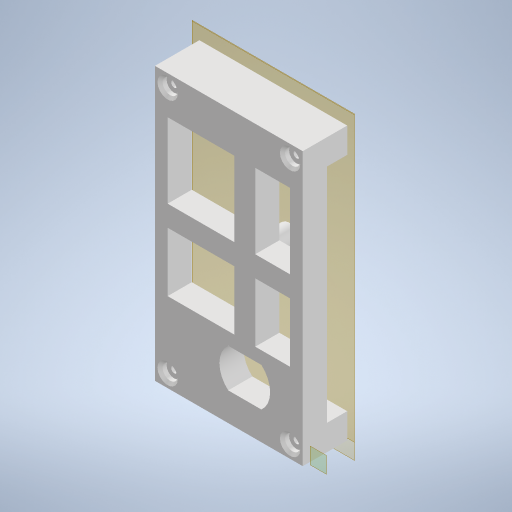
# Autodesk Inventor part: housingFront
Saved by Autodesk Inventor 2023 (Build 270158000, 158)
## iProperties
Created: 2023-03-11
Part Number: housingFront
Material: Generic
Document SubType Name: Modeling
Designer: shrey
Density: 1 g/cm^3
Appearance: Default
Author: shrey
Autodesk Inventor part; units mm, degrees
(part 1 of 2)
ref_plane "YZ Plane" through (0, 0, 0) normal (1, 0, 0) x (0, 1, 0)
ref_plane "XZ Plane" through (0, 0, 0) normal (0, 1, 0) x (-1, 0, 0)
ref_plane "XY Plane" through (0, 0, 0) normal (0, 0, 1) x (1, 0, 0)
ref_plane "Work Plane1" through (29.0854, -74.8946, 2) normal (0, 0, 1) x (1, 0, 0)
ref_plane "Work Plane2" through (29.0854, -80.3446, 2) normal (0, 0, 1) x (1, 0, 0)
sketch "Sketch3" plane through (29.0854, -80.3446, 2) normal (0, 0, 1) x (1, 0, 0)
  line L0 (29.0856, -48.6611) -> (29.0856, 58.6611) construction
  line L1 (29.0856, 58.6611) -> (-29.0856, 58.6611) construction
  line L2 (-29.0856, 58.6611) -> (-29.0856, -48.6611) construction
  line L3 (-29.0856, -48.6611) -> (29.0856, -48.6611) construction
  line L4 (29.0856, -48.6611) -> (-29.0856, -48.6611)
  line L5 (-29.0856, -48.6611) -> (-29.0856, 58.6611)
  line L6 (-29.0856, 58.6611) -> (29.0856, 58.6611)
  line L7 (29.0856, 58.6611) -> (29.0856, -48.6611)
  line L8 (29.0856, 48.6611) -> (-29.0856, 48.6611)
  spline S0 degree 3 poles (-74.8819, 38.2677) (-74.7621, 38.4578) (-74.5823, 38.743) (-74.3613, 39.1343) (-74.2025, 39.4317) (-74.052, 39.7333) (-73.9102, 40.0391) (-73.7782, 40.3493) (-73.6568, 40.6638) (-73.5477, 40.9828) (-73.4518, 41.306) (-73.3893, 41.58) (-73.3442, 41.8001) (-73.2966, 41.962) (-73.2322, 42.118) (-73.1482, 42.2647) (-73.0598, 42.3744) (-72.9799, 42.4536) (-72.9123, 42.5041) (-72.8431, 42.5525) (-72.7668, 42.5886) (-72.6893, 42.6221) (-72.6072, 42.6419) (-72.5245, 42.6586) (-72.4119, 42.6626) (-72.2715, 42.66) (-72.1312, 42.6626) (-72.0186, 42.6586) (-71.9359, 42.6419) (-71.8538, 42.6221) (-71.7763, 42.5886) (-71.7, 42.5525) (-71.6308, 42.5041) (-71.5632, 42.4536) (-71.4833, 42.3744) (-71.3948, 42.2647) (-71.3109, 42.118) (-71.2465, 41.962) (-71.1988, 41.8001) (-71.1538, 41.58) (-71.0913, 41.306) (-70.9954, 40.9828) (-70.8863, 40.6638) (-70.7649, 40.3493) (-70.6329, 40.0391) (-70.4911, 39.7333) (-70.3406, 39.4317) (-70.1818, 39.1343) (-69.9608, 38.743) (-69.781, 38.4578) (-69.6612, 38.2677) knots -1.0784 -1.0784 -1.0784 -1.0784 -1.010995 -0.977291 -0.943586 -0.909882 -0.876178 -0.842474 -0.80877 -0.775067 -0.741365 -0.707665 -0.690816 -0.67397 -0.657123 -0.640284 -0.623449 -0.615023 -0.606598 -0.598176 -0.589749 -0.581327 -0.572901 -0.564477 -0.556053 -0.5392 -0.522347 -0.513923 -0.505499 -0.497074 -0.488651 -0.480225 -0.471802 -0.463377 -0.454951 -0.438116 -0.421277 -0.40443 -0.387584 -0.370735 -0.337035 -0.303333 -0.26963 -0.235926 -0.202222 -0.168518 -0.134814 -0.101109 -0.067405 0 0 0 0 construction
  line L9 (-69.6612, 38.2677) -> (-68.5989, 38.2677) construction
  spline S1 degree 3 poles (-68.5989, 38.2677) (-68.4791, 38.4578) (-68.2993, 38.743) (-68.0783, 39.1343) (-67.9195, 39.4317) (-67.769, 39.7333) (-67.6272, 40.0391) (-67.4952, 40.3493) (-67.3738, 40.6638) (-67.2647, 40.9828) (-67.1688, 41.306) (-67.1063, 41.58) (-67.0612, 41.8001) (-67.0136, 41.962) (-66.9492, 42.118) (-66.8652, 42.2647) (-66.7768, 42.3744) (-66.6969, 42.4536) (-66.6293, 42.5041) (-66.5601, 42.5525) (-66.4838, 42.5886) (-66.4063, 42.6221) (-66.3242, 42.6419) (-66.2415, 42.6586) (-66.1289, 42.6626) (-65.9885, 42.66) (-65.8482, 42.6626) (-65.7356, 42.6586) (-65.6529, 42.6419) (-65.5708, 42.6221) (-65.4933, 42.5886) (-65.417, 42.5525) (-65.3478, 42.5041) (-65.2802, 42.4536) (-65.2003, 42.3744) (-65.1118, 42.2647) (-65.0279, 42.118) (-64.9635, 41.962) (-64.9158, 41.8001) (-64.8708, 41.58) (-64.8083, 41.306) (-64.7124, 40.9828) (-64.6033, 40.6638) (-64.4819, 40.3493) (-64.3499, 40.0391) (-64.2081, 39.7333) (-64.0576, 39.4317) (-63.8988, 39.1343) (-63.6778, 38.743) (-63.498, 38.4578) (-63.3782, 38.2677) knots -1.0784 -1.0784 -1.0784 -1.0784 -1.010995 -0.977291 -0.943586 -0.909882 -0.876178 -0.842474 -0.80877 -0.775067 -0.741365 -0.707665 -0.690816 -0.67397 -0.657123 -0.640284 -0.623449 -0.615023 -0.606598 -0.598176 -0.589749 -0.581327 -0.572901 -0.564477 -0.556053 -0.5392 -0.522347 -0.513923 -0.505499 -0.497074 -0.488651 -0.480225 -0.471802 -0.463377 -0.454951 -0.438116 -0.421277 -0.40443 -0.387584 -0.370735 -0.337035 -0.303333 -0.26963 -0.235926 -0.202222 -0.168518 -0.134814 -0.101109 -0.067405 0 0 0 0 construction
  line L10 (-63.3782, 38.2677) -> (-62.3159, 38.2677) construction
  spline S2 degree 3 poles (-62.3159, 38.2677) (-62.1961, 38.4578) (-62.0163, 38.743) (-61.7953, 39.1343) (-61.6365, 39.4317) (-61.486, 39.7333) (-61.3442, 40.0391) (-61.2122, 40.3493) (-61.0908, 40.6638) (-60.9817, 40.9828) (-60.8858, 41.306) (-60.8233, 41.58) (-60.7782, 41.8001) (-60.7306, 41.962) (-60.6662, 42.118) (-60.5822, 42.2647) (-60.4938, 42.3744) (-60.4139, 42.4536) (-60.3463, 42.5041) (-60.2771, 42.5525) (-60.2008, 42.5886) (-60.1233, 42.6221) (-60.0412, 42.6419) (-59.9585, 42.6586) (-59.8459, 42.6626) (-59.7055, 42.66) (-59.5652, 42.6626) (-59.4526, 42.6586) (-59.3699, 42.6419) (-59.2878, 42.6221) (-59.2103, 42.5886) (-59.134, 42.5525) (-59.0648, 42.5041) (-58.9972, 42.4536) (-58.9173, 42.3744) (-58.8288, 42.2647) (-58.7449, 42.118) (-58.6805, 41.962) (-58.6328, 41.8001) (-58.5878, 41.58) (-58.5253, 41.306) (-58.4294, 40.9828) (-58.3203, 40.6638) (-58.1989, 40.3493) (-58.0669, 40.0391) (-57.9251, 39.7333) (-57.7746, 39.4317) (-57.6158, 39.1343) (-57.3948, 38.743) (-57.215, 38.4578) (-57.0952, 38.2677) knots -1.0784 -1.0784 -1.0784 -1.0784 -1.010995 -0.977291 -0.943586 -0.909882 -0.876178 -0.842474 -0.80877 -0.775067 -0.741365 -0.707665 -0.690816 -0.67397 -0.657123 -0.640284 -0.623449 -0.615023 -0.606598 -0.598176 -0.589749 -0.581327 -0.572901 -0.564477 -0.556053 -0.5392 -0.522347 -0.513923 -0.505499 -0.497074 -0.488651 -0.480225 -0.471802 -0.463377 -0.454951 -0.438116 -0.421277 -0.40443 -0.387584 -0.370735 -0.337035 -0.303333 -0.26963 -0.235926 -0.202222 -0.168518 -0.134814 -0.101109 -0.067405 0 0 0 0 construction
  line L11 (-57.0952, 38.2677) -> (-56.0329, 38.2677) construction
  spline S3 degree 3 poles (-56.0329, 38.2677) (-55.9131, 38.4578) (-55.7333, 38.743) (-55.5123, 39.1343) (-55.3535, 39.4317) (-55.203, 39.7333) (-55.0612, 40.0391) (-54.9292, 40.3493) (-54.8078, 40.6638) (-54.6987, 40.9828) (-54.6028, 41.306) (-54.5403, 41.58) (-54.4952, 41.8001) (-54.4476, 41.962) (-54.3832, 42.118) (-54.2992, 42.2647) (-54.2108, 42.3744) (-54.1309, 42.4536) (-54.0633, 42.5041) (-53.9941, 42.5525) (-53.9178, 42.5886) (-53.8403, 42.6221) (-53.7582, 42.6419) (-53.6755, 42.6586) (-53.5629, 42.6626) (-53.4225, 42.66) (-53.2822, 42.6626) (-53.1696, 42.6586) (-53.0869, 42.6419) (-53.0048, 42.6221) (-52.9273, 42.5886) (-52.851, 42.5525) (-52.7818, 42.5041) (-52.7142, 42.4536) (-52.6343, 42.3744) (-52.5458, 42.2647) (-52.4619, 42.118) (-52.3975, 41.962) (-52.3498, 41.8001) (-52.3048, 41.58) (-52.2423, 41.306) (-52.1464, 40.9828) (-52.0373, 40.6638) (-51.9159, 40.3493) (-51.7839, 40.0391) (-51.6421, 39.7333) (-51.4916, 39.4317) (-51.3328, 39.1343) (-51.1118, 38.743) (-50.932, 38.4578) (-50.8122, 38.2677) knots -1.0784 -1.0784 -1.0784 -1.0784 -1.010995 -0.977291 -0.943586 -0.909882 -0.876178 -0.842474 -0.80877 -0.775067 -0.741365 -0.707665 -0.690816 -0.67397 -0.657123 -0.640284 -0.623449 -0.615023 -0.606598 -0.598176 -0.589749 -0.581327 -0.572901 -0.564477 -0.556053 -0.5392 -0.522347 -0.513923 -0.505499 -0.497074 -0.488651 -0.480225 -0.471802 -0.463377 -0.454951 -0.438116 -0.421277 -0.40443 -0.387584 -0.370735 -0.337035 -0.303333 -0.26963 -0.235926 -0.202222 -0.168518 -0.134814 -0.101109 -0.067405 0 0 0 0 construction
  line L12 (-50.8122, 38.2677) -> (-49.7499, 38.2677) construction
  spline S4 degree 3 poles (-49.7499, 38.2677) (-49.6301, 38.4578) (-49.4503, 38.743) (-49.2293, 39.1343) (-49.0705, 39.4317) (-48.92, 39.7333) (-48.7782, 40.0391) (-48.6462, 40.3493) (-48.5248, 40.6638) (-48.4157, 40.9828) (-48.3198, 41.306) (-48.2573, 41.58) (-48.2122, 41.8001) (-48.1646, 41.962) (-48.1002, 42.118) (-48.0162, 42.2647) (-47.9278, 42.3744) (-47.8479, 42.4536) (-47.7803, 42.5041) (-47.7111, 42.5525) (-47.6348, 42.5886) (-47.5573, 42.6221) (-47.4752, 42.6419) (-47.3925, 42.6586) (-47.2799, 42.6626) (-47.1395, 42.66) (-46.9992, 42.6626) (-46.8866, 42.6586) (-46.8039, 42.6419) (-46.7218, 42.6221) (-46.6443, 42.5886) (-46.568, 42.5525) (-46.4988, 42.5041) (-46.4312, 42.4536) (-46.3513, 42.3744) (-46.2628, 42.2647) (-46.1789, 42.118) (-46.1145, 41.962) (-46.0668, 41.8001) (-46.0218, 41.58) (-45.9593, 41.306) (-45.8634, 40.9828) (-45.7543, 40.6638) (-45.6329, 40.3493) (-45.5009, 40.0391) (-45.3591, 39.7333) (-45.2086, 39.4317) (-45.0498, 39.1343) (-44.8288, 38.743) (-44.649, 38.4578) (-44.5292, 38.2677) knots -1.0784 -1.0784 -1.0784 -1.0784 -1.010995 -0.977291 -0.943586 -0.909882 -0.876178 -0.842474 -0.80877 -0.775067 -0.741365 -0.707665 -0.690816 -0.67397 -0.657123 -0.640284 -0.623449 -0.615023 -0.606598 -0.598176 -0.589749 -0.581327 -0.572901 -0.564477 -0.556053 -0.5392 -0.522347 -0.513923 -0.505499 -0.497074 -0.488651 -0.480225 -0.471802 -0.463377 -0.454951 -0.438116 -0.421277 -0.40443 -0.387584 -0.370735 -0.337035 -0.303333 -0.26963 -0.235926 -0.202222 -0.168518 -0.134814 -0.101109 -0.067405 0 0 0 0 construction
  line L13 (-44.5292, 38.2677) -> (-43.4669, 38.2677) construction
  spline S5 degree 3 poles (-43.4669, 38.2677) (-43.3471, 38.4578) (-43.1673, 38.743) (-42.9463, 39.1343) (-42.7875, 39.4317) (-42.637, 39.7333) (-42.4952, 40.0391) (-42.3632, 40.3493) (-42.2418, 40.6638) (-42.1327, 40.9828) (-42.0368, 41.306) (-41.9743, 41.58) (-41.9292, 41.8001) (-41.8816, 41.962) (-41.8172, 42.118) (-41.7332, 42.2647) (-41.6448, 42.3744) (-41.5649, 42.4536) (-41.4973, 42.5041) (-41.4281, 42.5525) (-41.3518, 42.5886) (-41.2743, 42.6221) (-41.1922, 42.6419) (-41.1095, 42.6586) (-40.9969, 42.6626) (-40.8565, 42.66) (-40.7162, 42.6626) (-40.6036, 42.6586) (-40.5209, 42.6419) (-40.4388, 42.6221) (-40.3613, 42.5886) (-40.285, 42.5525) (-40.2158, 42.5041) (-40.1482, 42.4536) (-40.0683, 42.3744) (-39.9798, 42.2647) (-39.8959, 42.118) (-39.8315, 41.962) (-39.7838, 41.8001) (-39.7388, 41.58) (-39.6763, 41.306) (-39.5804, 40.9828) (-39.4713, 40.6638) (-39.3499, 40.3493) (-39.2179, 40.0391) (-39.0761, 39.7333) (-38.9256, 39.4317) (-38.7668, 39.1343) (-38.5458, 38.743) (-38.366, 38.4578) (-38.2462, 38.2677) knots -1.0784 -1.0784 -1.0784 -1.0784 -1.010995 -0.977291 -0.943586 -0.909882 -0.876178 -0.842474 -0.80877 -0.775067 -0.741365 -0.707665 -0.690816 -0.67397 -0.657123 -0.640284 -0.623449 -0.615023 -0.606598 -0.598176 -0.589749 -0.581327 -0.572901 -0.564477 -0.556053 -0.5392 -0.522347 -0.513923 -0.505499 -0.497074 -0.488651 -0.480225 -0.471802 -0.463377 -0.454951 -0.438116 -0.421277 -0.40443 -0.387584 -0.370735 -0.337035 -0.303333 -0.26963 -0.235926 -0.202222 -0.168518 -0.134814 -0.101109 -0.067405 0 0 0 0 construction
  line L14 (-38.2462, 38.2677) -> (-37.1839, 38.2677) construction
  spline S6 degree 3 poles (-37.1839, 38.2677) (-37.0641, 38.4578) (-36.8843, 38.743) (-36.6633, 39.1343) (-36.5045, 39.4317) (-36.354, 39.7333) (-36.2122, 40.0391) (-36.0802, 40.3493) (-35.9588, 40.6638) (-35.8497, 40.9828) (-35.7538, 41.306) (-35.6913, 41.58) (-35.6462, 41.8001) (-35.5986, 41.962) (-35.5342, 42.118) (-35.4502, 42.2647) (-35.3618, 42.3744) (-35.2819, 42.4536) (-35.2143, 42.5041) (-35.1451, 42.5525) (-35.0688, 42.5886) (-34.9913, 42.6221) (-34.9092, 42.6419) (-34.8265, 42.6586) (-34.7139, 42.6626) (-34.5735, 42.66) (-34.4332, 42.6626) (-34.3206, 42.6586) (-34.2379, 42.6419) (-34.1558, 42.6221) (-34.0783, 42.5886) (-34.002, 42.5525) (-33.9328, 42.5041) (-33.8652, 42.4536) (-33.7853, 42.3744) (-33.6968, 42.2647) (-33.6129, 42.118) (-33.5485, 41.962) (-33.5008, 41.8001) (-33.4558, 41.58) (-33.3933, 41.306) (-33.2974, 40.9828) (-33.1883, 40.6638) (-33.0669, 40.3493) (-32.9349, 40.0391) (-32.7931, 39.7333) (-32.6426, 39.4317) (-32.4838, 39.1343) (-32.2628, 38.743) (-32.083, 38.4578) (-31.9632, 38.2677) knots -1.0784 -1.0784 -1.0784 -1.0784 -1.010995 -0.977291 -0.943586 -0.909882 -0.876178 -0.842474 -0.80877 -0.775067 -0.741365 -0.707665 -0.690816 -0.67397 -0.657123 -0.640284 -0.623449 -0.615023 -0.606598 -0.598176 -0.589749 -0.581327 -0.572901 -0.564477 -0.556053 -0.5392 -0.522347 -0.513923 -0.505499 -0.497074 -0.488651 -0.480225 -0.471802 -0.463377 -0.454951 -0.438116 -0.421277 -0.40443 -0.387584 -0.370735 -0.337035 -0.303333 -0.26963 -0.235926 -0.202222 -0.168518 -0.134814 -0.101109 -0.067405 0 0 0 0 construction
  line L15 (-31.9632, 38.2677) -> (-30.9009, 38.2677) construction
  spline S7 degree 3 poles (-30.9009, 38.2677) (-30.7811, 38.4578) (-30.6013, 38.743) (-30.3803, 39.1343) (-30.2215, 39.4317) (-30.071, 39.7333) (-29.9292, 40.0391) (-29.7972, 40.3493) (-29.6758, 40.6638) (-29.5667, 40.9828) (-29.4708, 41.306) (-29.4083, 41.58) (-29.3632, 41.8001) (-29.3156, 41.962) (-29.2512, 42.118) (-29.1672, 42.2647) (-29.0788, 42.3744) (-28.9989, 42.4536) (-28.9313, 42.5041) (-28.8621, 42.5525) (-28.7858, 42.5886) (-28.7083, 42.6221) (-28.6262, 42.6419) (-28.5435, 42.6586) (-28.4309, 42.6626) (-28.2905, 42.66) (-28.1502, 42.6626) (-28.0376, 42.6586) (-27.9549, 42.6419) (-27.8728, 42.6221) (-27.7953, 42.5886) (-27.719, 42.5525) (-27.6498, 42.5041) (-27.5822, 42.4536) (-27.5023, 42.3744) (-27.4138, 42.2647) (-27.3299, 42.118) (-27.2655, 41.962) (-27.2178, 41.8001) (-27.1728, 41.58) (-27.1103, 41.306) (-27.0144, 40.9828) (-26.9053, 40.6638) (-26.7839, 40.3493) (-26.6519, 40.0391) (-26.5101, 39.7333) (-26.3596, 39.4317) (-26.2008, 39.1343) (-25.9798, 38.743) (-25.8, 38.4578) (-25.6802, 38.2677) knots -1.0784 -1.0784 -1.0784 -1.0784 -1.010995 -0.977291 -0.943586 -0.909882 -0.876178 -0.842474 -0.80877 -0.775067 -0.741365 -0.707665 -0.690816 -0.67397 -0.657123 -0.640284 -0.623449 -0.615023 -0.606598 -0.598176 -0.589749 -0.581327 -0.572901 -0.564477 -0.556053 -0.5392 -0.522347 -0.513923 -0.505499 -0.497074 -0.488651 -0.480225 -0.471802 -0.463377 -0.454951 -0.438116 -0.421277 -0.40443 -0.387584 -0.370735 -0.337035 -0.303333 -0.26963 -0.235926 -0.202222 -0.168518 -0.134814 -0.101109 -0.067405 0 0 0 0 construction
  line L16 (-25.6802, 38.2677) -> (-24.6179, 38.2677) construction
  spline S8 degree 3 poles (-24.6179, 38.2677) (-24.4981, 38.4578) (-24.3183, 38.743) (-24.0973, 39.1343) (-23.9385, 39.4317) (-23.788, 39.7333) (-23.6462, 40.0391) (-23.5142, 40.3493) (-23.3928, 40.6638) (-23.2837, 40.9828) (-23.1878, 41.306) (-23.1253, 41.58) (-23.0802, 41.8001) (-23.0326, 41.962) (-22.9682, 42.118) (-22.8842, 42.2647) (-22.7958, 42.3744) (-22.7159, 42.4536) (-22.6483, 42.5041) (-22.5791, 42.5525) (-22.5028, 42.5886) (-22.4253, 42.6221) (-22.3432, 42.6419) (-22.2605, 42.6586) (-22.1479, 42.6626) (-22.0075, 42.66) (-21.8672, 42.6626) (-21.7546, 42.6586) (-21.6719, 42.6419) (-21.5898, 42.6221) (-21.5123, 42.5886) (-21.436, 42.5525) (-21.3668, 42.5041) (-21.2992, 42.4536) (-21.2193, 42.3744) (-21.1308, 42.2647) (-21.0469, 42.118) (-20.9825, 41.962) (-20.9348, 41.8001) (-20.8898, 41.58) (-20.8273, 41.306) (-20.7314, 40.9828) (-20.6223, 40.6638) (-20.5009, 40.3493) (-20.3689, 40.0391) (-20.2271, 39.7333) (-20.0766, 39.4317) (-19.9178, 39.1343) (-19.6968, 38.743) (-19.517, 38.4578) (-19.3972, 38.2677) knots -1.0784 -1.0784 -1.0784 -1.0784 -1.010995 -0.977291 -0.943586 -0.909882 -0.876178 -0.842474 -0.80877 -0.775067 -0.741365 -0.707665 -0.690816 -0.67397 -0.657123 -0.640284 -0.623449 -0.615023 -0.606598 -0.598176 -0.589749 -0.581327 -0.572901 -0.564477 -0.556053 -0.5392 -0.522347 -0.513923 -0.505499 -0.497074 -0.488651 -0.480225 -0.471802 -0.463377 -0.454951 -0.438116 -0.421277 -0.40443 -0.387584 -0.370735 -0.337035 -0.303333 -0.26963 -0.235926 -0.202222 -0.168518 -0.134814 -0.101109 -0.067405 0 0 0 0 construction
  line L17 (-19.3972, 38.2677) -> (-18.3349, 38.2677) construction
  spline S9 degree 3 poles (-18.3349, 38.2677) (-18.2151, 38.4578) (-18.0353, 38.743) (-17.8143, 39.1343) (-17.6555, 39.4317) (-17.505, 39.7333) (-17.3632, 40.0391) (-17.2312, 40.3493) (-17.1098, 40.6638) (-17.0007, 40.9828) (-16.9048, 41.306) (-16.8423, 41.58) (-16.7972, 41.8001) (-16.7496, 41.962) (-16.6852, 42.118) (-16.6012, 42.2647) (-16.5128, 42.3744) (-16.4329, 42.4536) (-16.3653, 42.5041) (-16.2961, 42.5525) (-16.2198, 42.5886) (-16.1423, 42.6221) (-16.0602, 42.6419) (-15.9775, 42.6586) (-15.8649, 42.6626) (-15.7245, 42.66) (-15.5842, 42.6626) (-15.4716, 42.6586) (-15.3889, 42.6419) (-15.3068, 42.6221) (-15.2293, 42.5886) (-15.153, 42.5525) (-15.0838, 42.5041) (-15.0162, 42.4536) (-14.9363, 42.3744) (-14.8478, 42.2647) (-14.7639, 42.118) (-14.6995, 41.962) (-14.6518, 41.8001) (-14.6068, 41.58) (-14.5443, 41.306) (-14.4484, 40.9828) (-14.3393, 40.6638) (-14.2179, 40.3493) (-14.0859, 40.0391) (-13.9441, 39.7333) (-13.7936, 39.4317) (-13.6348, 39.1343) (-13.4138, 38.743) (-13.234, 38.4578) (-13.1142, 38.2677) knots -1.0784 -1.0784 -1.0784 -1.0784 -1.010995 -0.977291 -0.943586 -0.909882 -0.876178 -0.842474 -0.80877 -0.775067 -0.741365 -0.707665 -0.690816 -0.67397 -0.657123 -0.640284 -0.623449 -0.615023 -0.606598 -0.598176 -0.589749 -0.581327 -0.572901 -0.564477 -0.556053 -0.5392 -0.522347 -0.513923 -0.505499 -0.497074 -0.488651 -0.480225 -0.471802 -0.463377 -0.454951 -0.438116 -0.421277 -0.40443 -0.387584 -0.370735 -0.337035 -0.303333 -0.26963 -0.235926 -0.202222 -0.168518 -0.134814 -0.101109 -0.067405 0 0 0 0 construction
  line L18 (-13.1142, 38.2677) -> (-12.0519, 38.2677) construction
  spline S10 degree 3 poles (-12.0519, 38.2677) (-11.9321, 38.4578) (-11.7523, 38.743) (-11.5313, 39.1343) (-11.3725, 39.4317) (-11.222, 39.7333) (-11.0802, 40.0391) (-10.9482, 40.3493) (-10.8268, 40.6638) (-10.7177, 40.9828) (-10.6218, 41.306) (-10.5593, 41.58) (-10.5142, 41.8001) (-10.4666, 41.962) (-10.4022, 42.118) (-10.3182, 42.2647) (-10.2298, 42.3744) (-10.1499, 42.4536) (-10.0823, 42.5041) (-10.0131, 42.5525) (-9.9368, 42.5886) (-9.8593, 42.6221) (-9.7772, 42.6419) (-9.6945, 42.6586) (-9.5819, 42.6626) (-9.4415, 42.66) (-9.3012, 42.6626) (-9.1886, 42.6586) (-9.1059, 42.6419) (-9.0238, 42.6221) (-8.9463, 42.5886) (-8.87, 42.5525) (-8.8008, 42.5041) (-8.7332, 42.4536) (-8.6533, 42.3744) (-8.5648, 42.2647) (-8.4809, 42.118) (-8.4165, 41.962) (-8.3688, 41.8001) (-8.3238, 41.58) (-8.2613, 41.306) (-8.1654, 40.9828) (-8.0563, 40.6638) (-7.9349, 40.3493) (-7.8029, 40.0391) (-7.6611, 39.7333) (-7.5106, 39.4317) (-7.3518, 39.1343) (-7.1308, 38.743) (-6.951, 38.4578) (-6.8312, 38.2677) knots -1.0784 -1.0784 -1.0784 -1.0784 -1.010995 -0.977291 -0.943586 -0.909882 -0.876178 -0.842474 -0.80877 -0.775067 -0.741365 -0.707665 -0.690816 -0.67397 -0.657123 -0.640284 -0.623449 -0.615023 -0.606598 -0.598176 -0.589749 -0.581327 -0.572901 -0.564477 -0.556053 -0.5392 -0.522347 -0.513923 -0.505499 -0.497074 -0.488651 -0.480225 -0.471802 -0.463377 -0.454951 -0.438116 -0.421277 -0.40443 -0.387584 -0.370735 -0.337035 -0.303333 -0.26963 -0.235926 -0.202222 -0.168518 -0.134814 -0.101109 -0.067405 0 0 0 0 construction
  line L19 (-6.8312, 38.2677) -> (-5.7689, 38.2677) construction
  spline S11 degree 3 poles (-5.7689, 38.2677) (-5.6491, 38.4578) (-5.4693, 38.743) (-5.2483, 39.1343) (-5.0895, 39.4317) (-4.939, 39.7333) (-4.7972, 40.0391) (-4.6652, 40.3493) (-4.5438, 40.6638) (-4.4347, 40.9828) (-4.3388, 41.306) (-4.2763, 41.58) (-4.2312, 41.8001) (-4.1836, 41.962) (-4.1192, 42.118) (-4.0352, 42.2647) (-3.9468, 42.3744) (-3.8669, 42.4536) (-3.7993, 42.5041) (-3.7301, 42.5525) (-3.6538, 42.5886) (-3.5763, 42.6221) (-3.4942, 42.6419) (-3.4115, 42.6586) (-3.2989, 42.6626) (-3.1585, 42.66) (-3.0182, 42.6626) (-2.9056, 42.6586) (-2.8229, 42.6419) (-2.7408, 42.6221) (-2.6633, 42.5886) (-2.587, 42.5525) (-2.5178, 42.5041) (-2.4502, 42.4536) (-2.3703, 42.3744) (-2.2818, 42.2647) (-2.1979, 42.118) (-2.1335, 41.962) (-2.0858, 41.8001) (-2.0408, 41.58) (-1.9783, 41.306) (-1.8824, 40.9828) (-1.7733, 40.6638) (-1.6519, 40.3493) (-1.5199, 40.0391) (-1.3781, 39.7333) (-1.2276, 39.4317) (-1.0688, 39.1343) (-0.8478, 38.743) (-0.668, 38.4578) (-0.5482, 38.2677) knots -1.0784 -1.0784 -1.0784 -1.0784 -1.010995 -0.977291 -0.943586 -0.909882 -0.876178 -0.842474 -0.80877 -0.775067 -0.741365 -0.707665 -0.690816 -0.67397 -0.657123 -0.640284 -0.623449 -0.615023 -0.606598 -0.598176 -0.589749 -0.581327 -0.572901 -0.564477 -0.556053 -0.5392 -0.522347 -0.513923 -0.505499 -0.497074 -0.488651 -0.480225 -0.471802 -0.463377 -0.454951 -0.438116 -0.421277 -0.40443 -0.387584 -0.370735 -0.337035 -0.303333 -0.26963 -0.235926 -0.202222 -0.168518 -0.134814 -0.101109 -0.067405 0 0 0 0 construction
  line L20 (-0.5482, 38.2677) -> (0.5141, 38.2677) construction
  spline S12 degree 3 poles (0.5141, 38.2677) (0.6339, 38.4578) (0.8137, 38.743) (1.0347, 39.1343) (1.1935, 39.4317) (1.344, 39.7333) (1.4858, 40.0391) (1.6178, 40.3493) (1.7392, 40.6638) (1.8483, 40.9828) (1.9442, 41.306) (2.0067, 41.58) (2.0518, 41.8001) (2.0994, 41.962) (2.1638, 42.118) (2.2478, 42.2647) (2.3362, 42.3744) (2.4161, 42.4536) (2.4837, 42.5041) (2.5529, 42.5525) (2.6292, 42.5886) (2.7067, 42.6221) (2.7888, 42.6419) (2.8715, 42.6586) (2.9841, 42.6626) (3.1245, 42.66) (3.2648, 42.6626) (3.3774, 42.6586) (3.4601, 42.6419) (3.5422, 42.6221) (3.6197, 42.5886) (3.696, 42.5525) (3.7652, 42.5041) (3.8328, 42.4536) (3.9127, 42.3744) (4.0012, 42.2647) (4.0851, 42.118) (4.1495, 41.962) (4.1972, 41.8001) (4.2422, 41.58) (4.3047, 41.306) (4.4006, 40.9828) (4.5097, 40.6638) (4.6311, 40.3493) (4.7631, 40.0391) (4.9049, 39.7333) (5.0554, 39.4317) (5.2142, 39.1343) (5.4352, 38.743) (5.615, 38.4578) (5.7348, 38.2677) knots -1.0784 -1.0784 -1.0784 -1.0784 -1.010995 -0.977291 -0.943586 -0.909882 -0.876178 -0.842474 -0.80877 -0.775067 -0.741365 -0.707665 -0.690816 -0.67397 -0.657123 -0.640284 -0.623449 -0.615023 -0.606598 -0.598176 -0.589749 -0.581327 -0.572901 -0.564477 -0.556053 -0.5392 -0.522347 -0.513923 -0.505499 -0.497074 -0.488651 -0.480225 -0.471802 -0.463377 -0.454951 -0.438116 -0.421277 -0.40443 -0.387584 -0.370735 -0.337035 -0.303333 -0.26963 -0.235926 -0.202222 -0.168518 -0.134814 -0.101109 -0.067405 0 0 0 0 construction
  line L21 (5.7348, 38.2677) -> (6.7971, 38.2677) construction
  spline S13 degree 3 poles (6.7971, 38.2677) (6.9169, 38.4578) (7.0967, 38.743) (7.3177, 39.1343) (7.4765, 39.4317) (7.627, 39.7333) (7.7688, 40.0391) (7.9008, 40.3493) (8.0222, 40.6638) (8.1313, 40.9828) (8.2272, 41.306) (8.2897, 41.58) (8.3348, 41.8001) (8.3824, 41.962) (8.4468, 42.118) (8.5308, 42.2647) (8.6192, 42.3744) (8.6991, 42.4536) (8.7667, 42.5041) (8.8359, 42.5525) (8.9122, 42.5886) (8.9897, 42.6221) (9.0718, 42.6419) (9.1545, 42.6586) (9.2671, 42.6626) (9.4075, 42.66) (9.5478, 42.6626) (9.6604, 42.6586) (9.7431, 42.6419) (9.8252, 42.6221) (9.9027, 42.5886) (9.979, 42.5525) (10.0482, 42.5041) (10.1158, 42.4536) (10.1957, 42.3744) (10.2842, 42.2647) (10.3681, 42.118) (10.4325, 41.962) (10.4802, 41.8001) (10.5252, 41.58) (10.5877, 41.306) (10.6836, 40.9828) (10.7927, 40.6638) (10.9141, 40.3493) (11.0461, 40.0391) (11.1879, 39.7333) (11.3384, 39.4317) (11.4972, 39.1343) (11.7182, 38.743) (11.898, 38.4578) (12.0178, 38.2677) knots -1.0784 -1.0784 -1.0784 -1.0784 -1.010995 -0.977291 -0.943586 -0.909882 -0.876178 -0.842474 -0.80877 -0.775067 -0.741365 -0.707665 -0.690816 -0.67397 -0.657123 -0.640284 -0.623449 -0.615023 -0.606598 -0.598176 -0.589749 -0.581327 -0.572901 -0.564477 -0.556053 -0.5392 -0.522347 -0.513923 -0.505499 -0.497074 -0.488651 -0.480225 -0.471802 -0.463377 -0.454951 -0.438116 -0.421277 -0.40443 -0.387584 -0.370735 -0.337035 -0.303333 -0.26963 -0.235926 -0.202222 -0.168518 -0.134814 -0.101109 -0.067405 0 0 0 0 construction
  line L22 (12.0178, 38.2677) -> (13.0801, 38.2677) construction
  spline S14 degree 3 poles (13.0801, 38.2677) (13.1999, 38.4578) (13.3797, 38.743) (13.6007, 39.1343) (13.7595, 39.4317) (13.91, 39.7333) (14.0518, 40.0391) (14.1838, 40.3493) (14.3052, 40.6638) (14.4143, 40.9828) (14.5102, 41.306) (14.5727, 41.58) (14.6178, 41.8001) (14.6654, 41.962) (14.7298, 42.118) (14.8138, 42.2647) (14.9022, 42.3744) (14.9821, 42.4536) (15.0497, 42.5041) (15.1189, 42.5525) (15.1952, 42.5886) (15.2727, 42.6221) (15.3548, 42.6419) (15.4375, 42.6586) (15.5501, 42.6626) (15.6905, 42.66) (15.8308, 42.6626) (15.9434, 42.6586) (16.0261, 42.6419) (16.1082, 42.6221) (16.1857, 42.5886) (16.262, 42.5525) (16.3312, 42.5041) (16.3988, 42.4536) (16.4787, 42.3744) (16.5672, 42.2647) (16.6511, 42.118) (16.7155, 41.962) (16.7632, 41.8001) (16.8082, 41.58) (16.8707, 41.306) (16.9666, 40.9828) (17.0757, 40.6638) (17.1971, 40.3493) (17.3291, 40.0391) (17.4709, 39.7333) (17.6214, 39.4317) (17.7802, 39.1343) (18.0012, 38.743) (18.181, 38.4578) (18.3008, 38.2677) knots -1.0784 -1.0784 -1.0784 -1.0784 -1.010995 -0.977291 -0.943586 -0.909882 -0.876178 -0.842474 -0.80877 -0.775067 -0.741365 -0.707665 -0.690816 -0.67397 -0.657123 -0.640284 -0.623449 -0.615023 -0.606598 -0.598176 -0.589749 -0.581327 -0.572901 -0.564477 -0.556053 -0.5392 -0.522347 -0.513923 -0.505499 -0.497074 -0.488651 -0.480225 -0.471802 -0.463377 -0.454951 -0.438116 -0.421277 -0.40443 -0.387584 -0.370735 -0.337035 -0.303333 -0.26963 -0.235926 -0.202222 -0.168518 -0.134814 -0.101109 -0.067405 0 0 0 0 construction
  line L23 (18.3008, 38.2677) -> (19.3631, 38.2677) construction
  spline S15 degree 3 poles (19.3631, 38.2677) (19.6162, 38.6692) (20.1932, 39.5845) (20.9176, 41.5755) (20.8702, 41.9228) (21.1976, 42.4054) (21.3044, 42.4855) (21.4079, 42.5551) (21.5044, 42.6151) (21.798, 42.6737) (21.9339, 42.661) (22.1841, 42.6619) (22.2948, 42.6594) (22.5189, 42.5692) (22.6126, 42.5087) (22.7518, 42.3928) (22.8133, 42.3105) (22.9221, 42.1521) (22.978, 42.0242) (23.0746, 41.7075) (23.0901, 41.5466) (23.5668, 39.8295) (24.4081, 38.5465) (24.5838, 38.2677) knots 0 0 0 0 0.142394 0.142394 0.262557 0.262557 0.314666 0.314666 0.34653 0.34653 0.372217 0.372217 0.394622 0.394622 0.411062 0.411062 0.432958 0.432958 0.48678 0.48678 0.562983 0.562983 0.900876 0.900876 0.900876 0.900876 construction
  line L24 (24.5838, 38.2677) -> (24.5838, 47.6611) construction
  line L25 (24.5838, 47.6611) -> (-75.4162, 47.6611) construction
  line L26 (-75.4162, 47.6611) -> (-75.4162, 38.2677) construction
  line L27 (-75.4162, 38.2677) -> (-74.8819, 38.2677) construction
  arc A0 (-17.6491, 1.2756) -> (5.2752, -15.3798) centre (6.2752, 10.1006) ccw construction
  line L28 (-17.6491, 1.2756) -> (-5.8144, 5.1209) construction
  arc A1 (-5.8144, 5.1209) -> (5.2752, -2.9361) centre (6.2752, 10.1006) ccw construction
  line L29 (5.2752, -2.9361) -> (5.2752, -15.3798) construction
  line L30 (30.8175, 3.1777) -> (18.9828, 7.0231) construction
  arc A2 (18.9828, 7.0231) -> (14.747, 20.0597) centre (6.2752, 10.1006) ccw construction
  line L31 (14.747, 20.0597) -> (22.0612, 30.1268) construction
  arc A3 (30.8175, 3.1777) -> (22.0612, 30.1268) centre (6.2752, 10.1006) ccw construction
  line L32 (-9.5108, 30.1268) -> (-2.1966, 20.0597) construction
  arc A4 (-2.1966, 20.0597) -> (-6.4325, 7.0231) centre (6.2752, 10.1006) ccw construction
  line L33 (-6.4325, 7.0231) -> (-18.2671, 3.1777) construction
  arc A5 (-9.5108, 30.1268) -> (-18.2671, 3.1777) centre (6.2752, 10.1006) ccw construction
  circle A6 centre (6.2752, 10.1006) radius 11.075 construction
  line L34 (20.4432, 31.3024) -> (13.129, 21.2353) construction
  arc A7 (13.129, 21.2353) -> (-0.5786, 21.2353) centre (6.2752, 10.1006) ccw construction
  line L35 (-0.5786, 21.2353) -> (-7.8928, 31.3024) construction
  arc A8 (20.4432, 31.3024) -> (-7.8928, 31.3024) centre (6.2752, 10.1006) ccw construction
  line L36 (7.2752, -15.3798) -> (7.2752, -2.9361) construction
  arc A9 (7.2752, -2.9361) -> (18.3648, 5.1209) centre (6.2752, 10.1006) ccw construction
  line L37 (18.3648, 5.1209) -> (30.1995, 1.2756) construction
  arc A10 (7.2752, -15.3798) -> (30.1995, 1.2756) centre (6.2752, 10.1006) ccw construction
  spline S16 degree 3 poles (10.3529, -21.6386) (10.4306, -21.4277) (10.5471, -21.1114) (10.682, -20.6826) (10.7755, -20.3588) (10.86, -20.0325) (10.935, -19.7038) (10.9997, -19.373) (11.0531, -19.0401) (11.0934, -18.7055) (11.12, -18.3693) (11.1242, -18.0884) (11.1225, -17.8637) (11.1355, -17.6954) (11.166, -17.5294) (11.2176, -17.3685) (11.2814, -17.2428) (11.3431, -17.1487) (11.3987, -17.0853) (11.4563, -17.0236) (11.5234, -16.9723) (11.5922, -16.9235) (11.6684, -16.887) (11.7459, -16.8535) (11.8552, -16.8262) (11.993, -16.7995) (12.1297, -16.7678) (12.2407, -16.7483) (12.3251, -16.7475) (12.4095, -16.7498) (12.4923, -16.7664) (12.5744, -16.7859) (12.6521, -16.8189) (12.7287, -16.8542) (12.8234, -16.9151) (12.9327, -17.0039) (13.0453, -17.13) (13.1407, -17.2692) (13.221, -17.4176) (13.3109, -17.6236) (13.4289, -17.8785) (13.59, -18.1748) (13.763, -18.4641) (13.9471, -18.7465) (14.1408, -19.0224) (14.343, -19.2921) (14.5529, -19.5559) (14.7701, -19.8137) (15.0676, -20.1505) (15.3028, -20.3921) (15.4595, -20.5531) knots -1.0784 -1.0784 -1.0784 -1.0784 -1.010995 -0.977291 -0.943586 -0.909882 -0.876178 -0.842474 -0.80877 -0.775067 -0.741365 -0.707665 -0.690816 -0.67397 -0.657123 -0.640284 -0.623449 -0.615023 -0.606598 -0.598176 -0.589749 -0.581327 -0.572901 -0.564477 -0.556053 -0.5392 -0.522347 -0.513923 -0.505499 -0.497074 -0.488651 -0.480225 -0.471802 -0.463377 -0.454951 -0.438116 -0.421277 -0.40443 -0.387584 -0.370735 -0.337035 -0.303333 -0.26963 -0.235926 -0.202222 -0.168518 -0.134814 -0.101109 -0.067405 0 0 0 0 construction
  arc A11 (15.4595, -20.5531) -> (16.8627, -20.0972) centre (6.2752, 10.1006) ccw construction
  spline S17 degree 3 poles (16.8627, -20.0972) (16.8948, -19.8748) (16.9431, -19.5412) (16.9858, -19.0937) (17.01, -18.7575) (17.0248, -18.4208) (17.0299, -18.0837) (17.0243, -17.7467) (17.0073, -17.41) (16.9772, -17.0742) (16.9334, -16.7399) (16.879, -16.4642) (16.8307, -16.2448) (16.8084, -16.0775) (16.8038, -15.9088) (16.8208, -15.7406) (16.857, -15.6045) (16.8978, -15.4996) (16.939, -15.426) (16.9825, -15.3536) (17.0375, -15.2896) (17.0947, -15.2274) (17.1616, -15.176) (17.2304, -15.1271) (17.3316, -15.0776) (17.4609, -15.0229) (17.588, -14.9634) (17.6925, -14.9213) (17.7749, -14.9029) (17.8579, -14.8876) (17.9424, -14.8867) (18.0267, -14.8887) (18.1097, -14.9048) (18.1919, -14.9234) (18.2972, -14.9633) (18.4226, -15.0274) (18.5589, -15.1273) (18.6812, -15.2437) (18.7906, -15.3722) (18.9213, -15.5549) (19.0898, -15.7798) (19.3089, -16.0361) (19.5383, -16.2831) (19.7771, -16.521) (20.0239, -16.7507) (20.2778, -16.9724) (20.5379, -17.1868) (20.8039, -17.3938) (21.1651, -17.6614) (21.4453, -17.8488) (21.6321, -17.9737) knots -1.0784 -1.0784 -1.0784 -1.0784 -1.010995 -0.977291 -0.943586 -0.909882 -0.876178 -0.842474 -0.80877 -0.775067 -0.741365 -0.707665 -0.690816 -0.67397 -0.657123 -0.640284 -0.623449 -0.615023 -0.606598 -0.598176 -0.589749 -0.581327 -0.572901 -0.564477 -0.556053 -0.5392 -0.522347 -0.513923 -0.505499 -0.497074 -0.488651 -0.480225 -0.471802 -0.463377 -0.454951 -0.438116 -0.421277 -0.40443 -0.387584 -0.370735 -0.337035 -0.303333 -0.26963 -0.235926 -0.202222 -0.168518 -0.134814 -0.101109 -0.067405 0 0 0 0 construction
  arc A12 (21.6321, -17.9737) -> (22.9098, -17.236) centre (6.2752, 10.1006) ccw construction
  spline S18 degree 3 poles (22.9098, -17.236) (22.895, -17.0118) (22.8728, -16.6754) (22.8216, -16.2289) (22.7753, -15.895) (22.7198, -15.5625) (22.6547, -15.2318) (22.5792, -14.9033) (22.4926, -14.5775) (22.3933, -14.2553) (22.2809, -13.9374) (22.1704, -13.6791) (22.0775, -13.4745) (22.0209, -13.3155) (21.9813, -13.1514) (21.963, -12.9834) (21.9701, -12.8427) (21.9882, -12.7316) (22.0132, -12.6511) (22.0407, -12.5712) (22.0812, -12.4971) (22.1242, -12.4245) (22.179, -12.3602) (22.2361, -12.2981) (22.3248, -12.2287) (22.4399, -12.1482) (22.5519, -12.0637) (22.6453, -12.0007) (22.7221, -11.9656) (22.8001, -11.9334) (22.8825, -11.9149) (22.9655, -11.8993) (23.0499, -11.8978) (23.1343, -11.8989) (23.2455, -11.9161) (23.3815, -11.9528) (23.5357, -12.0221) (23.6795, -12.1105) (23.8132, -12.2134) (23.9791, -12.365) (24.1906, -12.5499) (24.4582, -12.7551) (24.7339, -12.949) (25.017, -13.1321) (25.3061, -13.3054) (25.6006, -13.4695) (25.8996, -13.6251) (26.2029, -13.7723) (26.6117, -13.959) (26.9248, -14.084) (27.1335, -14.1674) knots -1.0784 -1.0784 -1.0784 -1.0784 -1.010995 -0.977291 -0.943586 -0.909882 -0.876178 -0.842474 -0.80877 -0.775067 -0.741365 -0.707665 -0.690816 -0.67397 -0.657123 -0.640284 -0.623449 -0.615023 -0.606598 -0.598176 -0.589749 -0.581327 -0.572901 -0.564477 -0.556053 -0.5392 -0.522347 -0.513923 -0.505499 -0.497074 -0.488651 -0.480225 -0.471802 -0.463377 -0.454951 -0.438116 -0.421277 -0.40443 -0.387584 -0.370735 -0.337035 -0.303333 -0.26963 -0.235926 -0.202222 -0.168518 -0.134814 -0.101109 -0.067405 0 0 0 0 construction
  arc A13 (27.1335, -14.1674) -> (28.2299, -13.1801) centre (6.2752, 10.1006) ccw construction
  spline S19 degree 3 poles (28.2299, -13.1801) (28.1688, -12.9639) (28.0772, -12.6395) (27.9342, -12.2133) (27.8196, -11.8964) (27.6961, -11.5827) (27.5636, -11.2727) (27.4215, -10.9671) (27.269, -10.6664) (27.1049, -10.3719) (26.9289, -10.0843) (26.7671, -9.8546) (26.6337, -9.6738) (26.5453, -9.5301) (26.4725, -9.3778) (26.4196, -9.2173) (26.3973, -9.0782) (26.3919, -8.9657) (26.3996, -8.8818) (26.41, -8.7979) (26.4341, -8.7171) (26.4611, -8.637) (26.5013, -8.5628) (26.5443, -8.4901) (26.6166, -8.4038) (26.7124, -8.3012) (26.8044, -8.1952) (26.8827, -8.1142) (26.9505, -8.0639) (27.0201, -8.0162) (27.0969, -7.981) (27.1748, -7.9485) (27.2571, -7.9294) (27.3398, -7.913) (27.4522, -7.9066) (27.5928, -7.9142) (27.758, -7.95) (27.9171, -8.0066) (28.0693, -8.0795) (28.263, -8.1933) (28.5084, -8.3301) (28.8128, -8.4751) (29.1228, -8.6075) (29.4378, -8.7278) (29.7566, -8.8372) (30.0788, -8.9365) (30.4036, -9.0265) (30.7308, -9.1074) (31.1696, -9.205) (31.5018, -9.2622) (31.7233, -9.3004) knots -1.0784 -1.0784 -1.0784 -1.0784 -1.010995 -0.977291 -0.943586 -0.909882 -0.876178 -0.842474 -0.80877 -0.775067 -0.741365 -0.707665 -0.690816 -0.67397 -0.657123 -0.640284 -0.623449 -0.615023 -0.606598 -0.598176 -0.589749 -0.581327 -0.572901 -0.564477 -0.556053 -0.5392 -0.522347 -0.513923 -0.505499 -0.497074 -0.488651 -0.480225 -0.471802 -0.463377 -0.454951 -0.438116 -0.421277 -0.40443 -0.387584 -0.370735 -0.337035 -0.303333 -0.26963 -0.235926 -0.202222 -0.168518 -0.134814 -0.101109 -0.067405 0 0 0 0 construction
  arc A14 (31.7233, -9.3004) -> (32.5905, -8.1068) centre (6.2752, 10.1006) ccw construction
  spline S20 degree 3 poles (32.5905, -8.1068) (32.4857, -7.9079) (32.3287, -7.6097) (32.1003, -7.2226) (31.9222, -6.9364) (31.7362, -6.6552) (31.5422, -6.3795) (31.3396, -6.1101) (31.128, -5.8477) (30.9062, -5.5938) (30.6742, -5.3491) (30.4683, -5.158) (30.3002, -5.0089) (30.1838, -4.8867) (30.0809, -4.7529) (29.9958, -4.6069) (29.9451, -4.4754) (29.9164, -4.3666) (29.9065, -4.2829) (29.8992, -4.1987) (29.906, -4.1146) (29.9158, -4.0307) (29.9397, -3.9497) (29.9666, -3.8697) (30.0194, -3.7702) (30.0918, -3.65) (30.1597, -3.5271) (30.2195, -3.4316) (30.2753, -3.3683) (30.3335, -3.3072) (30.4013, -3.2568) (30.4707, -3.2088) (30.5472, -3.173) (30.6247, -3.1398) (30.7333, -3.1102) (30.8725, -3.0884) (31.0415, -3.0891) (31.2088, -3.1113) (31.3729, -3.151) (31.5861, -3.222) (31.8545, -3.3048) (32.1824, -3.3834) (32.5132, -3.4484) (32.8463, -3.5005) (33.1809, -3.5413) (33.5166, -3.5715) (33.8531, -3.5919) (34.19, -3.6031) (34.6394, -3.6073) (34.9763, -3.5942) (35.2008, -3.5855) knots -1.0784 -1.0784 -1.0784 -1.0784 -1.010995 -0.977291 -0.943586 -0.909882 -0.876178 -0.842474 -0.80877 -0.775067 -0.741365 -0.707665 -0.690816 -0.67397 -0.657123 -0.640284 -0.623449 -0.615023 -0.606598 -0.598176 -0.589749 -0.581327 -0.572901 -0.564477 -0.556053 -0.5392 -0.522347 -0.513923 -0.505499 -0.497074 -0.488651 -0.480225 -0.471802 -0.463377 -0.454951 -0.438116 -0.421277 -0.40443 -0.387584 -0.370735 -0.337035 -0.303333 -0.26963 -0.235926 -0.202222 -0.168518 -0.134814 -0.101109 -0.067405 0 0 0 0 construction
  arc A15 (35.2008, -3.5855) -> (35.8009, -2.2376) centre (6.2752, 10.1006) ccw construction
  spline S21 degree 3 poles (35.8009, -2.2376) (35.6572, -2.0649) (35.4415, -1.8058) (35.1376, -1.4747) (34.9039, -1.2318) (34.6635, -0.9954) (34.4165, -0.7661) (34.1623, -0.5447) (33.9007, -0.332) (33.631, -0.1298) (33.3532, 0.0614) (33.112, 0.2054) (32.9166, 0.3163) (32.7774, 0.4117) (32.6489, 0.5212) (32.5353, 0.6463) (32.4584, 0.7643) (32.4077, 0.8648) (32.3806, 0.9447) (32.3559, 1.0255) (32.3451, 1.1092) (32.3372, 1.1933) (32.3437, 1.2774) (32.3534, 1.3613) (32.3844, 1.4696) (32.4302, 1.6023) (32.4711, 1.7366) (32.5097, 1.8424) (32.5512, 1.9159) (32.5954, 1.9878) (32.6512, 2.0512) (32.7092, 2.1126) (32.7766, 2.1635) (32.8455, 2.2121) (32.9455, 2.2636) (33.0771, 2.3139) (33.2426, 2.3484) (33.4109, 2.3614) (33.5796, 2.3567) (33.8029, 2.3316) (34.0827, 2.3063) (34.4198, 2.2977) (34.7568, 2.3028) (35.0934, 2.3211) (35.4292, 2.3509) (35.7639, 2.3911) (36.0973, 2.4411) (36.4291, 2.5002) (36.8696, 2.5895) (37.1964, 2.6724) (37.4142, 2.7276) knots -1.0784 -1.0784 -1.0784 -1.0784 -1.010995 -0.977291 -0.943586 -0.909882 -0.876178 -0.842474 -0.80877 -0.775067 -0.741365 -0.707665 -0.690816 -0.67397 -0.657123 -0.640284 -0.623449 -0.615023 -0.606598 -0.598176 -0.589749 -0.581327 -0.572901 -0.564477 -0.556053 -0.5392 -0.522347 -0.513923 -0.505499 -0.497074 -0.488651 -0.480225 -0.471802 -0.463377 -0.454951 -0.438116 -0.421277 -0.40443 -0.387584 -0.370735 -0.337035 -0.303333 -0.26963 -0.235926 -0.202222 -0.168518 -0.134814 -0.101109 -0.067405 0 0 0 0 construction
  arc A16 (37.4142, 2.7276) -> (37.721, 4.1707) centre (6.2752, 10.1006) ccw construction
  spline S22 degree 3 poles (37.721, 4.1707) (37.5444, 4.3098) (37.2796, 4.5184) (36.9135, 4.7791) (36.6344, 4.9681) (36.3502, 5.1493) (36.0608, 5.3222) (35.7662, 5.486) (35.4661, 5.6396) (35.1602, 5.7814) (34.8488, 5.9106) (34.5829, 6.0013) (34.3687, 6.0692) (34.2127, 6.1335) (34.0642, 6.2139) (33.9271, 6.3127) (33.8273, 6.4121) (33.7568, 6.4999) (33.7137, 6.5724) (33.6728, 6.6463) (33.6448, 6.7259) (33.6196, 6.8065) (33.6085, 6.8902) (33.6005, 6.9742) (33.6083, 7.0866) (33.6256, 7.2259) (33.6377, 7.3658) (33.6534, 7.4773) (33.6787, 7.5578) (33.707, 7.6374) (33.7484, 7.711) (33.7923, 7.7831) (33.8477, 7.8469) (33.9049, 7.9088) (33.9921, 7.98) (34.1104, 8.0565) (34.2651, 8.1246) (34.427, 8.1724) (34.5929, 8.2028) (34.8166, 8.2247) (35.0955, 8.2582) (35.427, 8.3198) (35.7557, 8.3949) (36.0811, 8.4828) (36.4034, 8.5817) (36.7224, 8.6906) (37.0381, 8.8088) (37.3504, 8.9357) (37.7627, 9.1146) (38.0651, 9.2636) (38.2667, 9.3629) knots -1.0784 -1.0784 -1.0784 -1.0784 -1.010995 -0.977291 -0.943586 -0.909882 -0.876178 -0.842474 -0.80877 -0.775067 -0.741365 -0.707665 -0.690816 -0.67397 -0.657123 -0.640284 -0.623449 -0.615023 -0.606598 -0.598176 -0.589749 -0.581327 -0.572901 -0.564477 -0.556053 -0.5392 -0.522347 -0.513923 -0.505499 -0.497074 -0.488651 -0.480225 -0.471802 -0.463377 -0.454951 -0.438116 -0.421277 -0.40443 -0.387584 -0.370735 -0.337035 -0.303333 -0.26963 -0.235926 -0.202222 -0.168518 -0.134814 -0.101109 -0.067405 0 0 0 0 construction
  arc A17 (38.2667, 9.3629) -> (38.2667, 10.8382) centre (6.2752, 10.1006) ccw construction
  spline S23 degree 3 poles (38.2667, 10.8382) (38.0651, 10.9376) (37.7627, 11.0865) (37.3504, 11.2655) (37.0381, 11.3923) (36.7224, 11.5105) (36.4034, 11.6194) (36.0811, 11.7183) (35.7557, 11.8062) (35.427, 11.8813) (35.0955, 11.9429) (34.8166, 11.9764) (34.5929, 11.9983) (34.427, 12.0287) (34.2651, 12.0765) (34.1104, 12.1446) (33.9921, 12.2211) (33.9049, 12.2923) (33.8477, 12.3543) (33.7923, 12.418) (33.7484, 12.4901) (33.707, 12.5637) (33.6787, 12.6433) (33.6534, 12.7238) (33.6377, 12.8353) (33.6256, 12.9752) (33.6083, 13.1145) (33.6005, 13.2269) (33.6085, 13.3109) (33.6196, 13.3946) (33.6448, 13.4752) (33.6728, 13.5548) (33.7137, 13.6287) (33.7568, 13.7012) (33.8273, 13.789) (33.9271, 13.8884) (34.0642, 13.9872) (34.2127, 14.0676) (34.3687, 14.1319) (34.5829, 14.1998) (34.8488, 14.2905) (35.1602, 14.4197) (35.4661, 14.5615) (35.7662, 14.7151) (36.0608, 14.8789) (36.3502, 15.0518) (36.6344, 15.233) (36.9135, 15.422) (37.2796, 15.6827) (37.5444, 15.8913) (37.721, 16.0304) knots -1.0784 -1.0784 -1.0784 -1.0784 -1.010995 -0.977291 -0.943586 -0.909882 -0.876178 -0.842474 -0.80877 -0.775067 -0.741365 -0.707665 -0.690816 -0.67397 -0.657123 -0.640284 -0.623449 -0.615023 -0.606598 -0.598176 -0.589749 -0.581327 -0.572901 -0.564477 -0.556053 -0.5392 -0.522347 -0.513923 -0.505499 -0.497074 -0.488651 -0.480225 -0.471802 -0.463377 -0.454951 -0.438116 -0.421277 -0.40443 -0.387584 -0.370735 -0.337035 -0.303333 -0.26963 -0.235926 -0.202222 -0.168518 -0.134814 -0.101109 -0.067405 0 0 0 0 construction
  arc A18 (37.721, 16.0304) -> (37.4142, 17.4735) centre (6.2752, 10.1006) ccw construction
  spline S24 degree 3 poles (37.4142, 17.4735) (37.1964, 17.5288) (36.8696, 17.6116) (36.4291, 17.7009) (36.0973, 17.7601) (35.7639, 17.81) (35.4292, 17.8503) (35.0934, 17.88) (34.7568, 17.8983) (34.4198, 17.9034) (34.0827, 17.8948) (33.8029, 17.8695) (33.5796, 17.8444) (33.4109, 17.8397) (33.2426, 17.8527) (33.0771, 17.8872) (32.9455, 17.9375) (32.8455, 17.989) (32.7766, 18.0377) (32.7092, 18.0885) (32.6512, 18.1499) (32.5954, 18.2133) (32.5512, 18.2852) (32.5097, 18.3587) (32.4711, 18.4646) (32.4302, 18.5988) (32.3844, 18.7315) (32.3534, 18.8398) (32.3437, 18.9237) (32.3372, 19.0079) (32.3451, 19.0919) (32.3559, 19.1757) (32.3806, 19.2564) (32.4077, 19.3363) (32.4584, 19.4368) (32.5353, 19.5548) (32.6489, 19.68) (32.7774, 19.7894) (32.9166, 19.8848) (33.112, 19.9957) (33.3532, 20.1397) (33.631, 20.3309) (33.9007, 20.5332) (34.1623, 20.7458) (34.4165, 20.9672) (34.6635, 21.1965) (34.9039, 21.4329) (35.1376, 21.6758) (35.4415, 22.0069) (35.6572, 22.266) (35.8009, 22.4388) knots -1.0784 -1.0784 -1.0784 -1.0784 -1.010995 -0.977291 -0.943586 -0.909882 -0.876178 -0.842474 -0.80877 -0.775067 -0.741365 -0.707665 -0.690816 -0.67397 -0.657123 -0.640284 -0.623449 -0.615023 -0.606598 -0.598176 -0.589749 -0.581327 -0.572901 -0.564477 -0.556053 -0.5392 -0.522347 -0.513923 -0.505499 -0.497074 -0.488651 -0.480225 -0.471802 -0.463377 -0.454951 -0.438116 -0.421277 -0.40443 -0.387584 -0.370735 -0.337035 -0.303333 -0.26963 -0.235926 -0.202222 -0.168518 -0.134814 -0.101109 -0.067405 0 0 0 0 construction
  arc A19 (35.8009, 22.4388) -> (35.2008, 23.7866) centre (6.2752, 10.1006) ccw construction
  spline S25 degree 3 poles (35.2008, 23.7866) (34.9763, 23.7953) (34.6394, 23.8084) (34.19, 23.8042) (33.8531, 23.793) (33.5166, 23.7726) (33.1809, 23.7424) (32.8463, 23.7016) (32.5132, 23.6495) (32.1824, 23.5845) (31.8545, 23.5059) (31.5861, 23.4231) (31.3729, 23.3521) (31.2088, 23.3124) (31.0415, 23.2902) (30.8725, 23.2895) (30.7333, 23.3113) (30.6247, 23.3409) (30.5472, 23.3742) (30.4707, 23.4099) (30.4013, 23.4579) (30.3335, 23.5083) (30.2753, 23.5695) (30.2195, 23.6328) (30.1597, 23.7282) (30.0918, 23.8511) (30.0194, 23.9713) (29.9666, 24.0708) (29.9397, 24.1508) (29.9158, 24.2318) (29.906, 24.3157) (29.8992, 24.3998) (29.9065, 24.484) (29.9164, 24.5677) (29.9451, 24.6765) (29.9958, 24.808) (30.0809, 24.954) (30.1838, 25.0878) (30.3002, 25.21) (30.4683, 25.3591) (30.6742, 25.5502) (30.9062, 25.7949) (31.128, 26.0488) (31.3396, 26.3112) (31.5422, 26.5807) (31.7362, 26.8563) (31.9222, 27.1375) (32.1003, 27.4237) (32.3287, 27.8108) (32.4857, 28.109) (32.5905, 28.3079) knots -1.0784 -1.0784 -1.0784 -1.0784 -1.010995 -0.977291 -0.943586 -0.909882 -0.876178 -0.842474 -0.80877 -0.775067 -0.741365 -0.707665 -0.690816 -0.67397 -0.657123 -0.640284 -0.623449 -0.615023 -0.606598 -0.598176 -0.589749 -0.581327 -0.572901 -0.564477 -0.556053 -0.5392 -0.522347 -0.513923 -0.505499 -0.497074 -0.488651 -0.480225 -0.471802 -0.463377 -0.454951 -0.438116 -0.421277 -0.40443 -0.387584 -0.370735 -0.337035 -0.303333 -0.26963 -0.235926 -0.202222 -0.168518 -0.134814 -0.101109 -0.067405 0 0 0 0 construction
  arc A20 (32.5905, 28.3079) -> (31.7233, 29.5015) centre (6.2752, 10.1006) ccw construction
  spline S26 degree 3 poles (31.7233, 29.5015) (31.5018, 29.4633) (31.1696, 29.4061) (30.7308, 29.3085) (30.4036, 29.2276) (30.0788, 29.1376) (29.7566, 29.0383) (29.4378, 28.9289) (29.1228, 28.8087) (28.8128, 28.6763) (28.5084, 28.5312) (28.263, 28.3944) (28.0693, 28.2806) (27.9171, 28.2077) (27.758, 28.1512) (27.5928, 28.1153) (27.4522, 28.1077) (27.3398, 28.1141) (27.2571, 28.1305) (27.1748, 28.1496) (27.0969, 28.1821) (27.0201, 28.2173) (26.9505, 28.265) (26.8827, 28.3153) (26.8044, 28.3963) (26.7124, 28.5023) (26.6166, 28.6049) (26.5443, 28.6912) (26.5013, 28.7639) (26.4611, 28.8382) (26.4341, 28.9182) (26.41, 28.9991) (26.3996, 29.0829) (26.3919, 29.1669) (26.3973, 29.2793) (26.4196, 29.4184) (26.4725, 29.5789) (26.5453, 29.7312) (26.6337, 29.8749) (26.7671, 30.0557) (26.9289, 30.2854) (27.1049, 30.573) (27.269, 30.8675) (27.4215, 31.1682) (27.5636, 31.4738) (27.6961, 31.7838) (27.8196, 32.0975) (27.9342, 32.4145) (28.0772, 32.8406) (28.1688, 33.165) (28.2299, 33.3813) knots -1.0784 -1.0784 -1.0784 -1.0784 -1.010995 -0.977291 -0.943586 -0.909882 -0.876178 -0.842474 -0.80877 -0.775067 -0.741365 -0.707665 -0.690816 -0.67397 -0.657123 -0.640284 -0.623449 -0.615023 -0.606598 -0.598176 -0.589749 -0.581327 -0.572901 -0.564477 -0.556053 -0.5392 -0.522347 -0.513923 -0.505499 -0.497074 -0.488651 -0.480225 -0.471802 -0.463377 -0.454951 -0.438116 -0.421277 -0.40443 -0.387584 -0.370735 -0.337035 -0.303333 -0.26963 -0.235926 -0.202222 -0.168518 -0.134814 -0.101109 -0.067405 0 0 0 0 construction
  arc A21 (28.2299, 33.3813) -> (27.1335, 34.3685) centre (6.2752, 10.1006) ccw construction
  spline S27 degree 3 poles (27.1335, 34.3685) (26.9248, 34.2851) (26.6117, 34.1601) (26.2029, 33.9734) (25.8996, 33.8262) (25.6006, 33.6706) (25.3061, 33.5065) (25.017, 33.3332) (24.7339, 33.1501) (24.4582, 32.9562) (24.1906, 32.751) (23.9791, 32.5661) (23.8132, 32.4146) (23.6795, 32.3116) (23.5357, 32.2232) (23.3815, 32.1539) (23.2455, 32.1172) (23.1343, 32.1) (23.0499, 32.0989) (22.9655, 32.1005) (22.8825, 32.116) (22.8001, 32.1345) (22.7221, 32.1667) (22.6453, 32.2018) (22.5519, 32.2648) (22.4399, 32.3494) (22.3248, 32.4298) (22.2361, 32.4992) (22.179, 32.5613) (22.1242, 32.6256) (22.0812, 32.6982) (22.0407, 32.7723) (22.0132, 32.8522) (21.9882, 32.9327) (21.9701, 33.0438) (21.963, 33.1845) (21.9813, 33.3525) (22.0209, 33.5166) (22.0775, 33.6756) (22.1704, 33.8802) (22.2809, 34.1385) (22.3933, 34.4564) (22.4926, 34.7786) (22.5792, 35.1044) (22.6547, 35.4329) (22.7198, 35.7636) (22.7753, 36.0961) (22.8216, 36.43) (22.8728, 36.8766) (22.895, 37.2129) (22.9098, 37.4372) knots -1.0784 -1.0784 -1.0784 -1.0784 -1.010995 -0.977291 -0.943586 -0.909882 -0.876178 -0.842474 -0.80877 -0.775067 -0.741365 -0.707665 -0.690816 -0.67397 -0.657123 -0.640284 -0.623449 -0.615023 -0.606598 -0.598176 -0.589749 -0.581327 -0.572901 -0.564477 -0.556053 -0.5392 -0.522347 -0.513923 -0.505499 -0.497074 -0.488651 -0.480225 -0.471802 -0.463377 -0.454951 -0.438116 -0.421277 -0.40443 -0.387584 -0.370735 -0.337035 -0.303333 -0.26963 -0.235926 -0.202222 -0.168518 -0.134814 -0.101109 -0.067405 0 0 0 0 construction
  arc A22 (22.9098, 37.4372) -> (21.6321, 38.1748) centre (6.2752, 10.1006) ccw construction
  spline S28 degree 3 poles (21.6321, 38.1748) (21.4453, 38.0499) (21.1651, 37.8625) (20.8039, 37.5949) (20.5379, 37.3879) (20.2778, 37.1736) (20.0239, 36.9518) (19.7771, 36.7222) (19.5383, 36.4842) (19.3089, 36.2372) (19.0898, 35.9809) (18.9213, 35.7561) (18.7906, 35.5733) (18.6812, 35.4448) (18.5589, 35.3285) (18.4226, 35.2286) (18.2972, 35.1644) (18.1919, 35.1245) (18.1097, 35.1059) (18.0267, 35.0898) (17.9424, 35.0878) (17.8579, 35.0887) (17.7749, 35.104) (17.6925, 35.1224) (17.588, 35.1646) (17.4609, 35.224) (17.3316, 35.2787) (17.2304, 35.3282) (17.1616, 35.3771) (17.0947, 35.4286) (17.0375, 35.4907) (16.9825, 35.5547) (16.939, 35.6271) (16.8978, 35.7007) (16.857, 35.8056) (16.8208, 35.9417) (16.8038, 36.1099) (16.8084, 36.2786) (16.8307, 36.4459) (16.879, 36.6653) (16.9334, 36.941) (16.9772, 37.2753) (17.0073, 37.6111) (17.0243, 37.9478) (17.0299, 38.2848) (17.0248, 38.6219) (17.01, 38.9586) (16.9858, 39.2948) (16.9431, 39.7423) (16.8948, 40.0759) (16.8627, 40.2983) knots -1.0784 -1.0784 -1.0784 -1.0784 -1.010995 -0.977291 -0.943586 -0.909882 -0.876178 -0.842474 -0.80877 -0.775067 -0.741365 -0.707665 -0.690816 -0.67397 -0.657123 -0.640284 -0.623449 -0.615023 -0.606598 -0.598176 -0.589749 -0.581327 -0.572901 -0.564477 -0.556053 -0.5392 -0.522347 -0.513923 -0.505499 -0.497074 -0.488651 -0.480225 -0.471802 -0.463377 -0.454951 -0.438116 -0.421277 -0.40443 -0.387584 -0.370735 -0.337035 -0.303333 -0.26963 -0.235926 -0.202222 -0.168518 -0.134814 -0.101109 -0.067405 0 0 0 0 construction
  arc A23 (16.8627, 40.2983) -> (15.4595, 40.7542) centre (6.2752, 10.1006) ccw construction